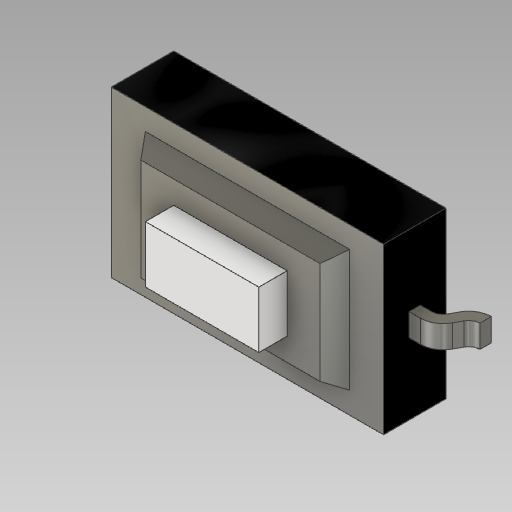
# Autodesk Inventor part: Switch
Saved by Autodesk Inventor 2020 (Build 240168000, 168)
## iProperties
Created: 2018-09-30
Part Number: Switch
Material: Generic
Document SubType Name: Modeling
Designer: amsmi
Density: 1 g/cm^3
Appearance: Default
Author: amsmi
Autodesk Inventor part; units mm, degrees
ref_plane "YZ Plane" through (0, 0, 0) normal (1, 0, 0) x (0, 1, 0)
ref_plane "XZ Plane" through (0, 0, 0) normal (0, 1, 0) x (-1, 0, 0)
sketch "Sketch1" plane through (0, 0, 0) normal (0, 0, 1) x (1, 0, 0)
  line L0 (3.048, -1.8479) -> (-3.048, -1.8479)
  line L1 (-3.048, -1.8479) -> (-3.048, 1.8478)
  line L2 (-3.048, 1.8478) -> (3.048, 1.8478)
  line L3 (3.048, 1.8478) -> (3.048, -1.8479)
  line L4 (3.048, -1.8479) -> (-3.048, 1.8478) construction
  line L5 (-3.048, -1.8479) -> (3.048, 1.8478) construction
  point P0 (0, 0)
  dimension "d0" = 6.096
  dimension "d1" = 3.6957
  constraints: 12 end point, 2 midpoint, 2 parallel, 1 horizontal, 1 perpendicular
  measures "d0" distance of L1.end L2.end
  measures "d1" distance of L0.end L1.end
extrude "Extrusion1" add sketch "Sketch1" along normal blind 1.397
sketch "Sketch2" plane through (0, 0, 1.397) normal (0, 0, 1) x (1, 0, 0)
  line L0 (2.286, 1.3653) -> (-2.286, 1.3653)
  line L1 (-2.286, 1.3653) -> (-2.286, -1.3653)
  line L2 (-2.286, -1.3653) -> (2.286, -1.3653)
  line L3 (2.286, -1.3653) -> (2.286, 1.3653)
  line L4 (2.286, 1.3653) -> (-2.286, -1.3653) construction
  line L5 (-2.286, 1.3653) -> (2.286, -1.3653) construction
  point P0 (0, 0)
  dimension "d4" = 4.572
  dimension "d5" = 2.7305
  constraints: 12 end point, 2 midpoint, 2 parallel, 1 horizontal, 1 perpendicular
  measures "d4" distance of L2.end L1.end
  measures "d5" distance of L1.end L0.end
ref_plane "Work Plane1" through (0, 0, 1.778) normal (0, 0, 1) x (1, 0, 0)
sketch "Sketch3" plane through (0, 0, 1.778) normal (0, 0, 1) x (1, 0, 0)
  line L0 (2.0066, 1.143) -> (-2.0066, 1.143)
  line L1 (-2.0066, 1.143) -> (-2.0066, -1.143)
  line L2 (-2.0066, -1.143) -> (2.0066, -1.143)
  line L3 (2.0066, -1.143) -> (2.0066, 1.143)
  line L4 (2.0066, 1.143) -> (-2.0066, -1.143) construction
  line L5 (-2.0066, 1.143) -> (2.0066, -1.143) construction
  point P0 (0, 0)
  dimension "d7" = 4.0132
  dimension "d8" = 2.286
  constraints: 12 end point, 2 midpoint, 2 parallel, 1 horizontal, 1 perpendicular
  measures "d7" distance of L2.end L1.end
  measures "d8" distance of L1.end L0.end
loft "Loft1" add profiles "Sketch2", "Sketch3"
sketch "Sketch4" plane through (-2.0066, 1.143, 1.778) normal (0, 0, 1) x (1, 0, 0)
  line L0 (3.2766, -0.508) -> (0.7366, -0.508)
  line L1 (0.7366, -0.508) -> (0.7366, -1.778)
  line L2 (0.7366, -1.778) -> (3.2766, -1.778)
  line L3 (3.2766, -1.778) -> (3.2766, -0.508)
  line L4 (3.2766, -0.508) -> (0.7366, -1.778) construction
  line L5 (0.7366, -0.508) -> (3.2766, -1.778) construction
  point P0 (2.0066, -1.143)
  dimension "d13" = 2.54
  dimension "d14" = 1.27
  constraints: 12 end point, 2 midpoint, 2 parallel, 1 horizontal, 1 perpendicular
  measures "d13" distance of L2.end L1.end
  measures "d14" distance of L1.end L0.end
extrude "Extrusion2" add sketch "Sketch4" along normal blind 0.635
sketch "Sketch5" plane through (0, 0, 0) normal (0, 1, 0) x (-1, 0, 0)
  line L0 (-3.048, 0) -> (-3.048, 1.397) construction
  line L1 (-3.048, 0.6985) -> (-3.302, 0.6985)
  arc A0 (-3.302, 0.6985) -> (-3.6382, 0.4968) centre (-3.302, 0.3175) ccw
  line L2 (-3.6382, 0.4968) -> (-3.7278, 0.3287)
  arc A1 (-4.064, 0.127) -> (-3.7278, 0.3287) centre (-4.064, 0.508) ccw
  line L3 (3.048, 0) -> (-3.048, 0) projected
  point P0 (0, 0)
  dimension "d17" = 1.016
  dimension "d18" = 0.127
  dimension "d19" = 0.254
  dimension "d20" = 0.381
  constraints: 4 end point, 4 point on circle, 3 tangent, 2 centre point, 1 equal radius, 1 horizontal, 1 midpoint, 1 vertical alignment
  measures "d17" distance from line of L0 A1.start
  measures "d18" distance from line of L3 A1.start
  measures "d19" distance of L1.start L1.end
  measures "d20" radius of A0
sketch "Sketch6" plane through (3.048, -1.8479, 0) normal (1, 0, 0) x (0, 0, -1)
  line L0 (0, 0) -> (-1.397, 0) projected
  line L1 (-1.397, 0) -> (-1.397, 3.6957) projected
  line L2 (-0.8255, 2.1019) -> (-0.5715, 2.1019)
  line L3 (-0.5715, 2.1019) -> (-0.5715, 1.5939)
  line L4 (-0.5715, 1.5939) -> (-0.8255, 1.5939)
  line L5 (-0.8255, 1.5939) -> (-0.8255, 2.1019)
  line L6 (-0.8255, 2.1019) -> (-0.5715, 1.5939) construction
  line L7 (-0.5715, 2.1019) -> (-0.8255, 1.5939) construction
  point P0 (0, 1.8479)
  point P1 (-0.6985, 1.8479)
  point P2 (-0.6985, 1.8479)
  point P3 (-0.6985, 1.8479)
  dimension "d21" = 0.254
  dimension "d22" = 0.508
  constraints: 12 end point, 2 midpoint, 2 parallel, 1 horizontal, 1 perpendicular
  measures "d21" distance of L3.end L4.end
  measures "d22" distance of L2.end L3.end
sweep "Sweep1" add profiles "Sketch6" path "Sketch5" path curves L1 A0 L2 A1
mirror "Mirror1" about plane through (0, 0, 0) normal (1, 0, 0) of "Sweep1"
body "Solid1"
